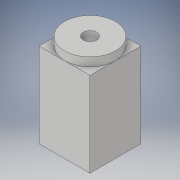
# Autodesk Inventor part: Troncox1
Saved by Autodesk Inventor 2019 (Build 230136000, 136)
## iProperties
Created: 2018-08-28
Part Number: Troncox1
Material: Genérico
Document SubType Name: Modeling
Designer: Cecilia Barrera Vill
Density: 1 g/cm^3
Appearance: Valor por defecto
Author: Cecilia Barrera Vill
Autodesk Inventor part; units mm, degrees
ref_plane "YZ Plane" through (0, 0, 0) normal (1, 0, 0) x (0, 1, 0)
ref_plane "XZ Plane" through (0, 0, 0) normal (0, 1, 0) x (-1, 0, 0)
ref_plane "XY Plane" through (0, 0, 0) normal (0, 0, 1) x (1, 0, 0)
sketch "Boceto1" plane through (0, 0, 0) normal (0, 1, 0) x (-1, 0, 0)
  line L0 (0, 0) -> (30, 0)
  line L1 (30, 0) -> (30, -30)
  line L2 (30, -30) -> (0, -30)
  line L3 (0, -30) -> (0, 0)
  circle A0 centre (15, -15) radius 4
  dimension "d0" = 30
  dimension "d1" = 30
  dimension "d2" = 8
  constraints: 8 end point, 2 parallel, 1 centre point, 1 horizontal, 1 perpendicular
  measures "d0" distance of L1.end L2.end
  measures "d1" distance of L0.end L1.end
  measures "d2" diameter of A0
extrude "Extrusión1" add sketch "Boceto1" along normal blind 50
sketch "Boceto2" plane through (0, 50, 0) normal (0, 1, 0) x (1, 0, 0)
  circle A0 centre (-15, 15) radius 4 projected
  circle A1 centre (-15, 15) radius 15
  point P0 (0, 0)
  dimension "d5" = 30
  constraints: 1 centre point, 1 coincident
  measures "d5" diameter of A1
extrude "Extrusión2" add sketch "Boceto2" along normal blind 5
sketch "Boceto3" plane through (0, 0, 0) normal (0, -1, 0) x (1, 0, 0)
  circle A0 centre (-15, -15) radius 4 projected
  circle A1 centre (-15, -15) radius 5.5
  line L0 (-2, -28) -> (-28, -28)
  line L1 (-28, -28) -> (-28, -2)
  line L2 (-28, -2) -> (-2, -2)
  line L3 (-2, -2) -> (-2, -28)
  line L4 (-2, -28) -> (-28, -2) construction
  line L5 (-28, -28) -> (-2, -2) construction
  point P0 (0, 0)
  dimension "d8" = 11
  dimension "d9" = 26
  dimension "d10" = 26
  constraints: 12 end point, 2 midpoint, 2 parallel, 1 centre point, 1 coincident, 1 horizontal, 1 perpendicular
  measures "d8" diameter of A1
  measures "d9" distance of L1.end L2.end
  measures "d10" distance of L0.end L1.end
extrude "Extrusión3" cut sketch "Boceto3" against normal blind 46 contours L0 L1 L2 L3
